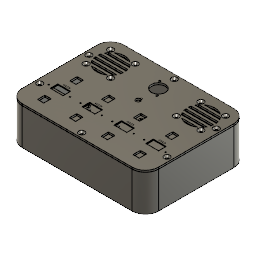
basestation_v3 (Autodesk Fusion 360 design; units mm, degrees)
Autodesk Fusion 360 part; units mm, degrees
note: some values were not read from the file. Chosen so that the rebuilt part matches the saved one: which face or edge a step refers to. Set by a fixed rule: which sketch regions a step uses.
(part 1 of 2)
sketch "Enclosure_main" plane through (0, 0, 0) normal (0, 1, 0) x (1, 0, 0)
  line L0 (0, 0) -> (230, 0)
  line L1 (230, 0) -> (230, -170)
  line L2 (230, -170) -> (0, -170)
  line L3 (0, -170) -> (0, 0)
  line L4 (0, -80) -> (10, -80)
  line L5 (10, -80) -> (10, -90)
  line L6 (10, -90) -> (0, -90)
  line L7 (0, -90) -> (0, -80)
  line L8 (0, -85) -> (230, -85) construction
  line L9 (115, 0) -> (115, -170) construction
  line L10 (5, -80) -> (5, -90) construction
  line L11 (0, -85) -> (10, -85) construction
  circle A0 centre (5, -85) radius 2.3
  line L12 (110, -10) -> (120, -10)
  line L13 (120, -10) -> (120, 0)
  line L14 (120, 0) -> (110, 0)
  line L15 (110, 0) -> (110, -10)
  line L16 (110, -5) -> (120, -5) construction
  line L17 (115, 0) -> (115, -10) construction
  circle A1 centre (115, -5) radius 2.3
  line L18 (220, -90) -> (230, -90)
  line L19 (230, -90) -> (230, -80)
  line L20 (230, -80) -> (220, -80)
  line L21 (220, -80) -> (220, -90)
  line L22 (225, -80) -> (225, -90) construction
  line L23 (220, -85) -> (230, -85) construction
  circle A2 centre (225, -85) radius 2.3
  line L24 (110, -170) -> (120, -170)
  line L25 (120, -170) -> (120, -160)
  line L26 (120, -160) -> (110, -160)
  line L27 (110, -160) -> (110, -170)
  line L28 (110, -165) -> (120, -165) construction
  line L29 (115, -170) -> (115, -160) construction
  circle A3 centre (115, -165) radius 2.3
  line L30 (20, -0.5) -> (76, -0.5) construction
  line L31 (76, -0.5) -> (76, -85.5) construction
  line L32 (76, -85.5) -> (20, -85.5) construction
  line L33 (20, -85.5) -> (20, -0.5) construction
  circle A4 centre (23.15, -3.65) radius 3
  circle A5 centre (23.15, -3.65) radius 1
  circle A6 centre (72.85, -3.65) radius 3
  circle A7 centre (72.85, -3.65) radius 1
  circle A8 centre (23.15, -61.65) radius 3
  circle A9 centre (72.85, -61.65) radius 3
  circle A10 centre (72.85, -61.65) radius 1
  circle A11 centre (23.15, -61.65) radius 1
  line L34 (181.9, -5) -> (181.9, -50) construction
  line L35 (181.9, -50) -> (151, -50) construction
  line L36 (151, -50) -> (151, -5) construction
  line L37 (151, -5) -> (181.9, -5) construction
  circle A12 centre (178.45, -46.55) radius 3
  circle A13 centre (154.45, -46.55) radius 3
  circle A14 centre (166.45, -10.3) radius 3
  circle A15 centre (166.45, -10.3) radius 1
  circle A16 centre (154.45, -46.55) radius 1
  circle A17 centre (178.45, -46.55) radius 1
  line L38 (79, -5) -> (99, -5) construction
  line L39 (99, -5) -> (99, -40) construction
  line L40 (99, -40) -> (79, -40) construction
  line L41 (79, -40) -> (79, -5) construction
  circle A18 centre (89, -8.9) radius 3
  circle A19 centre (89, -36.1) radius 3
  circle A20 centre (89, -36.1) radius 1
  circle A21 centre (89, -8.9) radius 1
  line L42 (78, -44.9949) -> (99.6, -45.0051) construction
  line L43 (99.6, -45.0051) -> (99.561, -75.7193) construction
  line L44 (99.561, -75.7193) -> (78, -76.2949) construction
  line L45 (78, -76.2949) -> (78, -44.9949) construction
  line L46 (88.8, -45) -> (88.7805, -76.0071) construction
  circle A22 centre (88.782, -73.6571) radius 3
  circle A23 centre (88.7985, -47.35) radius 3
  circle A24 centre (88.782, -73.6571) radius 1
  circle A25 centre (88.7985, -47.35) radius 1
  line L47 (166.45, -5) -> (166.45, -50) construction
  line L48 (0, -37.5) -> (10, -37.5)
  line L49 (10, -37.5) -> (10, -47.5)
  line L50 (10, -47.5) -> (0, -47.5)
  line L51 (0, -47.5) -> (0, -37.5)
  line L52 (0, -42.5) -> (10, -42.5) construction
  line L53 (5, -37.5) -> (5, -47.5) construction
  circle A26 centre (5, -42.5) radius 2.3
  line L54 (0, -122.5) -> (10, -122.5)
  line L55 (10, -122.5) -> (10, -132.5)
  line L56 (10, -132.5) -> (0, -132.5)
  line L57 (0, -132.5) -> (0, -122.5)
  line L58 (0, -127.5) -> (10, -127.5) construction
  line L59 (5, -122.5) -> (5, -132.5) construction
  circle A27 centre (5, -127.5) radius 2.3
  line L60 (220, -122.5) -> (230, -122.5)
  line L61 (230, -122.5) -> (230, -132.5)
  line L62 (230, -132.5) -> (220, -132.5)
  line L63 (220, -132.5) -> (220, -122.5)
  line L64 (220, -127.5) -> (230, -127.5) construction
  line L65 (225, -122.5) -> (225, -132.5) construction
  circle A28 centre (225, -127.5) radius 2.3
  line L66 (220, -37.5) -> (230, -37.5)
  line L67 (230, -37.5) -> (230, -47.5)
  line L68 (230, -47.5) -> (220, -47.5)
  line L69 (220, -47.5) -> (220, -37.5)
  line L70 (220, -42.5) -> (230, -42.5) construction
  line L71 (225, -37.5) -> (225, -47.5) construction
  circle A29 centre (225, -42.5) radius 2.3
  dimension "d1" = 170
  dimension "d2" = 230
  dimension "d282" = 10
  dimension "d283" = 10
  dimension "d284" = 4.6
  dimension "d307" = 10
  dimension "d308" = 10
  dimension "d309" = 4.6
  dimension "d310" = 10
  dimension "d311" = 10
  dimension "d312" = 4.6
  dimension "d313" = 10
  dimension "d314" = 10
  dimension "d315" = 4.6
  dimension "d349" = 56
  dimension "d350" = 85
  dimension "d351" = 20
  dimension "d352" = 0.5
  dimension "d353" = 6
  dimension "d354" = 2
  dimension "d355" = 3.15
  dimension "d356" = 3.15
  dimension "d357" = 6
  dimension "d358" = 3.15
  dimension "d359" = 3.15
  dimension "d360" = 2
  dimension "d361" = 6
  dimension "d362" = 3.15
  dimension "d363" = 58
  dimension "d364" = 6
  dimension "d365" = 3.15
  dimension "d366" = 58
  dimension "d367" = 2
  dimension "d368" = 2
  dimension "d369" = 45
  dimension "d370" = 30.9
  dimension "d371" = 6
  dimension "d372" = 6
  dimension "d373" = 6
  dimension "d375" = 3.45
  dimension "d376" = 3.45
  dimension "d377" = 3.45
  dimension "d378" = 3.45
  dimension "d379" = 2
  dimension "d380" = 2
  dimension "d381" = 2
  dimension "d384" = 20
  dimension "d385" = 35
  dimension "d386" = 6
  dimension "d387" = 10
  dimension "d388" = 3.9
  dimension "d389" = 6
  dimension "d390" = 10
  dimension "d391" = 3.9
  dimension "d392" = 2
  dimension "d393" = 2
  dimension "d394" = 5
  dimension "d395" = 3
  dimension "d396" = 21.6
  dimension "d397" = 31.3
  dimension "d398" = 6
  dimension "d399" = 6
  dimension "d402" = 2
  dimension "d403" = 2
  dimension "d469" = 5
  dimension "d470" = 75
  dimension "d471" = 5.3
  dimension "d484" = 10
  dimension "d485" = 10
  dimension "d486" = 4.6
  dimension "d487" = 42.5
  dimension "d488" = 10
  dimension "d489" = 10
  dimension "d490" = 4.6
  dimension "d491" = 42.5
  dimension "d492" = 10
  dimension "d493" = 10
  dimension "d494" = 4.6
  dimension "d495" = 42.5
  dimension "d496" = 10
  dimension "d497" = 10
  dimension "d498" = 42.5
  dimension "d499" = 4.6
  dimension "d517" = 2
  dimension "d518" = 2.35
  dimension "d519" = 2.35
  dimension "d520" = 5
  measures "d282" distance of L0.start
  measures "d284" diameter of A0
  measures "d308" distance of L0.start
  measures "d309" diameter of A1
  measures "d312" diameter of A2
  measures "d315" diameter of A3
  measures "d351" distance of L3 L33
  measures "d352" distance of L0 L30
  measures "d353" diameter of A4
  measures "d354" diameter of A5
  measures "d357" diameter of A6
  measures "d360" diameter of A7
  measures "d361" diameter of A8
  measures "d363" distance of L0.start
  measures "d364" diameter of A9
  measures "d366" distance of L0.start
  measures "d367" diameter of A10
  measures "d368" diameter of A11
  measures "d371" diameter of A12
  measures "d372" diameter of A13
  measures "d373" diameter of A14
  measures "d376" distance of L36 L0.start
  measures "d377" distance of L35 L3.end L0
  measures "d378" distance of L34 L3.end L0
  measures "d379" diameter of A15
  measures "d380" diameter of A16
  measures "d381" diameter of A17
  measures "d385" distance of L0.start
  measures "d386" diameter of A18
  measures "d387" distance of L41
  measures "d388" distance of L38
  measures "d389" diameter of A19
  measures "d390" distance of L41 L0.start
  measures "d392" diameter of A20
  measures "d393" diameter of A21
  measures "d394" distance of L0 L38
  measures "d395" distance of L31 L41
  measures "d398" diameter of A22
  measures "d399" diameter of A23
  measures "d402" diameter of A24 L1
  measures "d403" diameter of A25
  measures "d469" distance of L0 L37
  measures "d470" distance of L31 L36
  measures "d484" distance of L0.start
  measures "d486" diameter of A26
  measures "d488" distance of L0.start
  measures "d490" diameter of A27
  measures "d494" diameter of A28
  measures "d497" distance of L3.end origin L0
  measures "d499" diameter of A29
  measures "d517" distance of L31 L45
extrude "Extrude1" add sketch "Enclosure_main" along normal blind 60 contours L0 L1 L2 L3 L4 L5 L6 L12 L13 L15 L18 L20 L21 L25 L26 L27 L48 L49 L50 L54 L55 L56 L60 L62 L63 L66 L68 L69 | L0 L12 L13 L14 L15 | L3 L48 L49 L50 L51 | L3 L4 L5 L6 L7 | L1 L66 L67 L68 L69 | L3 L54 L55 L56 L57 | L1 L18 L19 L20 L21 | L1 L60 L61 L62 L63 | L2 L24 L25 L26 L27 | A0 | A1 | A2 | A3 | A4 | A5 | A6 | A7 | A8 | A9 | A10 | A11 | A12 | A13 | A14 | A15 | A16 | A17 | A18 | A19 | A20 | A21 | A22 | A23 | A24 | A25 | A26 | A27 | A28 | A29 makes body 1
fillet "Fillet1" radius 20 4 edges at (230, 30, 170) (0, 30, 170) (230, 30, 0) (0, 30, 0) on bodies 1
shell "Shell1" thickness 3 outward yes removed faces 0 bodies 1
ref_plane "WorkPlane1" through (115, 60, 85) normal (0, 1, 0) x (0, 0, 1)
split "Split1" by plane through (115, 60, 85) normal (0, 1, 0) bodies 1 makes body 2 at (83.3333, 63, 114.3333)
sketch "Enclosure_upper" plane through (0, 63, 0) normal (0, 1, 0) x (-1, 0, 0)
  arc A0 (-20, -3) -> (3, 20) centre (-20, 20) ccw
  line L0 (3, 20) -> (3, 150)
  arc A1 (3, 150) -> (-20, 173) centre (-20, 150) ccw
  line L1 (-20, 173) -> (-210, 173)
  arc A2 (-210, 173) -> (-233, 150) centre (-210, 150) ccw
  line L2 (-233, 150) -> (-233, 20)
  arc A3 (-233, 20) -> (-210, -3) centre (-210, 20) ccw
  line L3 (-210, -3) -> (-20, -3)
  line L4 (3, 85) -> (-233, 85) construction
  line L5 (-115, -3) -> (-115, 173) construction
  line L6 (-10.25, 10.25) -> (-63.75, 10.25) construction
  line L7 (-63.75, 10.25) -> (-63.75, 63.75) construction
  line L8 (-63.75, 63.75) -> (-10.25, 63.75) construction
  line L9 (-10.25, 63.75) -> (-10.25, 10.25) construction
  line L10 (-37, 10.25) -> (-37, 63.75) construction
  line L11 (-10.25, 37) -> (-63.75, 37) construction
  circle A4 centre (-37, 37) radius 24
  circle A5 centre (-15.75, 15.75) radius 2
  circle A6 centre (-58.25, 15.75) radius 2
  circle A7 centre (-58.25, 58.25) radius 2
  circle A8 centre (-15.75, 58.25) radius 2
  line L12 (-10.25, 13) -> (-63.75, 13)
  line L13 (-63.75, 13) -> (-63.75, 17.8)
  line L14 (-63.75, 17.8) -> (-10.25, 17.8)
  line L15 (-10.25, 17.8) -> (-10.25, 13)
  line L16 (-10.25, 17.8) -> (-63.75, 17.8)
  line L17 (-166.25, 13) -> (-219.75, 13)
  circle A9 centre (-171.75, 15.75) radius 2
  line L18 (-219.75, 17.8) -> (-166.25, 17.8)
  line L19 (-219.75, 13) -> (-219.75, 17.8)
  line L20 (-166.25, 17.8) -> (-219.75, 17.8)
  circle A10 centre (-214.25, 58.25) radius 2
  circle A11 centre (-171.75, 58.25) radius 2
  circle A12 centre (-214.25, 15.75) radius 2
  line L21 (-166.25, 17.8) -> (-166.25, 13)
  line L22 (-219.75, 10.25) -> (-219.75, 63.75) construction
  line L23 (-219.75, 63.75) -> (-166.25, 63.75) construction
  line L24 (-166.25, 10.25) -> (-219.75, 10.25) construction
  circle A13 centre (-193, 37) radius 24
  line L25 (-166.25, 63.75) -> (-166.25, 10.25) construction
  line L26 (-193, 10.25) -> (-193, 63.75) construction
  line L27 (-102, 17) -> (-128, 17) construction
  line L28 (-128, 17) -> (-128, 48) construction
  line L29 (-128, 48) -> (-102, 48) construction
  line L30 (-102, 48) -> (-102, 17) construction
  line L31 (-102, 32.5) -> (-128, 32.5) construction
  line L32 (-115, 17) -> (-115, 48) construction
  circle A14 centre (-115, 32.5) radius 12.15
  circle A15 centre (-105.2, 20.4) radius 1.6
  circle A16 centre (-124.8, 44.6) radius 1.6
  circle A17 centre (-115, 67.5) radius 5.75 construction
  circle A18 centre (-115, 67.5) radius 4
  line L33 (-113.5, 60.75) -> (-116.5, 60.75)
  line L34 (-116.5, 60.75) -> (-116.5, 62.75)
  line L35 (-116.5, 62.75) -> (-113.5, 62.75)
  line L36 (-113.5, 62.75) -> (-113.5, 60.75)
  line L37 (-113.5, 61.75) -> (-116.5, 61.75) construction
  line L38 (-115, 62.75) -> (-115, 60.75) construction
  line L39 (-10.25, 22.12) -> (-63.75, 22.12)
  line L40 (-10.25, 17.32) -> (-63.75, 17.32)
  line L41 (-10.25, 26.44) -> (-63.75, 26.44)
  line L42 (-10.25, 21.64) -> (-63.75, 21.64)
  line L43 (-10.25, 30.76) -> (-63.75, 30.76)
  line L44 (-10.25, 25.96) -> (-63.75, 25.96)
  line L45 (-10.25, 35.08) -> (-63.75, 35.08)
  line L46 (-10.25, 30.28) -> (-63.75, 30.28)
  line L47 (-10.25, 39.4) -> (-63.75, 39.4)
  line L48 (-10.25, 34.6) -> (-63.75, 34.6)
  line L49 (-10.25, 43.72) -> (-63.75, 43.72)
  line L50 (-10.25, 38.92) -> (-63.75, 38.92)
  line L51 (-10.25, 48.04) -> (-63.75, 48.04)
  line L52 (-10.25, 43.24) -> (-63.75, 43.24)
  line L53 (-10.25, 52.36) -> (-63.75, 52.36)
  line L54 (-10.25, 47.56) -> (-63.75, 47.56)
  line L55 (-10.25, 56.68) -> (-63.75, 56.68)
  line L56 (-10.25, 51.88) -> (-63.75, 51.88)
  line L57 (-10.25, 61) -> (-63.75, 61)
  line L58 (-10.25, 56.2) -> (-63.75, 56.2)
  line L59 (-166.25, 37) -> (-219.75, 37) construction
  line L60 (-166.25, 22.12) -> (-219.75, 22.12)
  line L61 (-166.25, 17.32) -> (-219.75, 17.32)
  line L62 (-166.25, 26.44) -> (-219.75, 26.44)
  line L63 (-166.25, 21.64) -> (-219.75, 21.64)
  line L64 (-166.25, 30.76) -> (-219.75, 30.76)
  line L65 (-166.25, 25.96) -> (-219.75, 25.96)
  line L66 (-166.25, 35.08) -> (-219.75, 35.08)
  line L67 (-166.25, 30.28) -> (-219.75, 30.28)
  line L68 (-166.25, 39.4) -> (-219.75, 39.4)
  line L69 (-166.25, 34.6) -> (-219.75, 34.6)
  line L70 (-166.25, 43.72) -> (-219.75, 43.72)
  line L71 (-166.25, 38.92) -> (-219.75, 38.92)
  line L72 (-166.25, 48.04) -> (-219.75, 48.04)
  line L73 (-166.25, 43.24) -> (-219.75, 43.24)
  line L74 (-166.25, 52.36) -> (-219.75, 52.36)
  line L75 (-166.25, 47.56) -> (-219.75, 47.56)
  line L76 (-166.25, 56.68) -> (-219.75, 56.68)
  line L77 (-166.25, 51.88) -> (-219.75, 51.88)
  line L78 (-166.25, 61) -> (-219.75, 61)
  line L79 (-166.25, 56.2) -> (-219.75, 56.2)
  line L80 (-27.15, 85) -> (-37.85, 85)
  line L81 (-37.85, 85) -> (-37.85, 97.7)
  line L82 (-37.85, 97.7) -> (-27.15, 97.7)
  line L83 (-27.15, 97.7) -> (-27.15, 85)
  line L84 (-27.15, 91.35) -> (-37.85, 91.35) construction
  line L85 (-32.5, 85) -> (-32.5, 97.7) construction
  line L86 (-18.5, 106.9) -> (-46.5, 106.9)
  line L87 (-46.5, 106.9) -> (-46.5, 135.4)
  line L88 (-46.5, 135.4) -> (-18.5, 135.4)
  line L89 (-18.5, 135.4) -> (-18.5, 106.9)
  line L90 (-18.5, 121.15) -> (-46.5, 121.15) construction
  line L91 (-32.5, 106.9) -> (-32.5, 135.4) construction
  line L92 (-21.5, 112.7) -> (-43.5, 112.7)
  line L93 (-43.5, 112.7) -> (-43.5, 125.7)
  line L94 (-43.5, 125.7) -> (-21.5, 125.7)
  line L95 (-21.5, 125.7) -> (-21.5, 112.7)
  line L96 (-27.15, 140.7) -> (-37.85, 140.7)
  line L97 (-37.85, 140.7) -> (-37.85, 153.4)
  line L98 (-37.85, 153.4) -> (-27.15, 153.4)
  line L99 (-27.15, 153.4) -> (-27.15, 140.7)
  line L100 (-32.5, 140.7) -> (-32.5, 153.4) construction
  line L101 (-27.15, 147.05) -> (-37.7784, 147.05) construction
  line L102 (-47, 117.25) -> (-54.8, 117.25)
  line L103 (-54.8, 117.25) -> (-54.8, 125.05)
  line L104 (-54.8, 125.05) -> (-47, 125.05)
  line L105 (-47, 125.05) -> (-47, 117.25)
  line L106 (-50.9, 117.25) -> (-50.9, 125.05) construction
  line L107 (-54.8, 121.15) -> (-47, 121.15) construction
  circle A19 centre (-50.9, 121.15) radius 1.6
  circle A20 centre (-50.9, 121.15) radius 1
  line L108 (-18, 117.25) -> (-10.2, 117.25)
  line L109 (-10.2, 117.25) -> (-10.2, 125.05)
  line L110 (-10.2, 125.05) -> (-18, 125.05)
  line L111 (-18, 125.05) -> (-18, 117.25)
  line L112 (-14.1, 117.25) -> (-14.1, 125.05) construction
  line L113 (-10.2, 121.15) -> (-18, 121.15) construction
  circle A21 centre (-14.1, 121.15) radius 1.6
  circle A22 centre (-14.1, 121.15) radius 1
  line L114 (-19, 107.4) -> (-24.5, 107.4)
  line L115 (-24.5, 107.4) -> (-24.5, 110.15)
  line L116 (-24.5, 110.15) -> (-19, 110.15)
  line L117 (-19, 110.15) -> (-19, 107.4)
  line L118 (-40.5, 107.4) -> (-46, 107.4)
  line L119 (-46, 107.4) -> (-46, 110.15)
  line L120 (-46, 110.15) -> (-40.5, 110.15)
  line L121 (-40.5, 110.15) -> (-40.5, 107.4)
  line L122 (-27.15, 107.4) -> (-37.85, 107.4)
  line L123 (-37.85, 107.4) -> (-37.85, 109.4)
  line L124 (-37.85, 109.4) -> (-27.15, 109.4)
  line L125 (-27.15, 109.4) -> (-27.15, 107.4)
  line L126 (-40.5, 132.15) -> (-46, 132.15)
  line L127 (-46, 132.15) -> (-46, 134.9)
  line L128 (-46, 134.9) -> (-40.5, 134.9)
  line L129 (-40.5, 134.9) -> (-40.5, 132.15)
  line L130 (-19, 132.15) -> (-24.5, 132.15)
  line L131 (-24.5, 132.15) -> (-24.5, 134.9)
  line L132 (-24.5, 134.9) -> (-19, 134.9)
  line L133 (-19, 134.9) -> (-19, 132.15)
  line L134 (-10.2, 117.25) -> (-54.8, 117.25)
  line L135 (-54.8, 117.25) -> (-54.8, 125.05)
  line L136 (-54.8, 125.05) -> (-10.2, 125.05)
  line L137 (-10.2, 125.05) -> (-10.2, 117.25)
  line L138 (-65.2, 125.05) -> (-73, 125.05)
  line L139 (-82.15, 91.35) -> (-92.85, 91.35) construction
  line L140 (-82.15, 107.4) -> (-92.85, 107.4)
  line L141 (-98.5, 125.7) -> (-76.5, 125.7)
  line L142 (-92.85, 85) -> (-92.85, 97.7)
  line L143 (-92.85, 107.4) -> (-92.85, 109.4)
  line L144 (-82.15, 109.4) -> (-82.15, 107.4)
  line L145 (-105.9, 117.25) -> (-105.9, 125.05) construction
  line L146 (-76.5, 125.7) -> (-76.5, 112.7)
  circle A23 centre (-105.9, 121.15) radius 1
  line L147 (-79.5, 134.9) -> (-74, 134.9)
  line L148 (-73, 117.25) -> (-65.2, 117.25)
  line L149 (-65.2, 117.25) -> (-65.2, 125.05)
  line L150 (-69.1, 117.25) -> (-69.1, 125.05) construction
  line L151 (-102, 117.25) -> (-109.8, 117.25)
  line L152 (-102, 125.05) -> (-102, 117.25)
  circle A24 centre (-105.9, 121.15) radius 1.6
  line L153 (-74, 132.15) -> (-79.5, 132.15)
  circle A25 centre (-69.1, 121.15) radius 1
  line L154 (-65.2, 125.05) -> (-65.2, 117.25)
  line L155 (-73, 125.05) -> (-73, 117.25)
  line L156 (-74, 134.9) -> (-74, 132.15)
  line L157 (-87.5, 85) -> (-87.5, 97.7) construction
  line L158 (-79.5, 110.15) -> (-74, 110.15)
  line L159 (-92.85, 109.4) -> (-82.15, 109.4)
  line L160 (-79.5, 132.15) -> (-79.5, 134.9)
  line L161 (-65.2, 121.15) -> (-73, 121.15) construction
  circle A26 centre (-69.1, 121.15) radius 1.6
  line L162 (-95.5, 132.15) -> (-101, 132.15)
  line L163 (-95.5, 134.9) -> (-95.5, 132.15)
  line L164 (-109.8, 121.15) -> (-102, 121.15) construction
  line L165 (-109.8, 125.05) -> (-102, 125.05)
  line L166 (-65.2, 117.25) -> (-109.8, 117.25)
  line L167 (-87.5, 106.9) -> (-87.5, 135.4) construction
  line L168 (-95.5, 107.4) -> (-101, 107.4)
  line L169 (-82.15, 140.7) -> (-92.85, 140.7)
  line L170 (-101, 107.4) -> (-101, 110.15)
  line L171 (-101, 110.15) -> (-95.5, 110.15)
  line L172 (-73, 106.4) -> (-102, 106.4)
  line L173 (-76.5, 112.7) -> (-98.5, 112.7)
  line L174 (-74, 107.4) -> (-79.5, 107.4)
  line L175 (-98.5, 112.7) -> (-98.5, 125.7)
  line L176 (-95.5, 110.15) -> (-95.5, 107.4)
  line L177 (-79.5, 107.4) -> (-79.5, 110.15)
  line L178 (-73, 135.9) -> (-73, 106.4)
  line L179 (-102, 135.9) -> (-73, 135.9)
  line L180 (-82.15, 153.4) -> (-82.15, 140.7)
  line L181 (-82.15, 147.05) -> (-92.7784, 147.05) construction
  line L182 (-73.5, 121.15) -> (-101.5, 121.15) construction
  line L183 (-92.85, 153.4) -> (-82.15, 153.4)
  line L184 (-101.5, 135.4) -> (-73.5, 135.4)
  line L185 (-73.5, 106.9) -> (-101.5, 106.9)
  line L186 (-92.85, 140.7) -> (-92.85, 153.4)
  line L187 (-87.5, 140.7) -> (-87.5, 153.4) construction
  line L188 (-109.8, 125.05) -> (-65.2, 125.05)
  line L189 (-73.5, 135.4) -> (-73.5, 106.9)
  line L190 (-102, 106.4) -> (-102, 135.9)
  line L191 (-101.5, 106.9) -> (-101.5, 135.4)
  line L192 (-109.8, 117.25) -> (-109.8, 125.05)
  line L193 (-109.8, 117.25) -> (-109.8, 125.05)
  line L194 (-74, 110.15) -> (-74, 107.4)
  line L195 (-82.15, 85) -> (-92.85, 85)
  line L196 (-101, 134.9) -> (-95.5, 134.9)
  line L197 (-82.15, 97.7) -> (-82.15, 85)
  line L198 (-92.85, 97.7) -> (-82.15, 97.7)
  line L199 (-101, 132.15) -> (-101, 134.9)
  line L200 (-137.15, 91.35) -> (-147.85, 91.35) construction
  line L201 (-156, 110.15) -> (-150.5, 110.15)
  line L202 (-131.5, 125.7) -> (-131.5, 112.7)
  line L203 (-147.85, 97.7) -> (-137.15, 97.7)
  line L204 (-128, 117.25) -> (-120.2, 117.25)
  line L205 (-137.15, 97.7) -> (-137.15, 85)
  line L206 (-137.15, 107.4) -> (-147.85, 107.4)
  line L207 (-147.85, 107.4) -> (-147.85, 109.4)
  line L208 (-147.85, 109.4) -> (-137.15, 109.4)
  line L209 (-147.85, 153.4) -> (-137.15, 153.4)
  line L210 (-142.5, 140.7) -> (-142.5, 153.4) construction
  line L211 (-150.5, 134.9) -> (-150.5, 132.15)
  line L212 (-150.5, 132.15) -> (-156, 132.15)
  line L213 (-147.85, 85) -> (-147.85, 97.7)
  line L214 (-142.5, 106.9) -> (-142.5, 135.4) construction
  line L215 (-120.2, 117.25) -> (-120.2, 125.05)
  line L216 (-128, 135.9) -> (-128, 106.4)
  line L217 (-150.5, 107.4) -> (-156, 107.4)
  line L218 (-137.15, 85) -> (-147.85, 85)
  line L219 (-150.5, 110.15) -> (-150.5, 107.4)
  line L220 (-128.5, 121.15) -> (-156.5, 121.15) construction
  line L221 (-156.5, 135.4) -> (-128.5, 135.4)
  line L222 (-147.85, 140.7) -> (-147.85, 153.4)
  line L223 (-153.5, 112.7) -> (-153.5, 125.7)
  line L224 (-128.5, 135.4) -> (-128.5, 106.9)
  line L225 (-156, 134.9) -> (-150.5, 134.9)
  line L226 (-142.5, 85) -> (-142.5, 97.7) construction
  line L227 (-124.1, 117.25) -> (-124.1, 125.05) construction
  line L228 (-134.5, 134.9) -> (-129, 134.9)
  line L229 (-164.8, 125.05) -> (-120.2, 125.05)
  line L230 (-128.5, 106.9) -> (-156.5, 106.9)
  line L231 (-120.2, 125.05) -> (-128, 125.05)
  line L232 (-157, 106.4) -> (-157, 135.9)
  line L233 (-156, 132.15) -> (-156, 134.9)
  line L234 (-164.8, 117.25) -> (-164.8, 125.05)
  line L235 (-164.8, 125.05) -> (-157, 125.05)
  line L236 (-164.8, 121.15) -> (-157, 121.15) construction
  line L237 (-120.2, 117.25) -> (-164.8, 117.25)
  line L238 (-153.5, 125.7) -> (-131.5, 125.7)
  line L239 (-160.9, 117.25) -> (-160.9, 125.05) construction
  line L240 (-137.15, 153.4) -> (-137.15, 140.7)
  line L241 (-128, 106.4) -> (-157, 106.4)
  line L242 (-137.15, 147.05) -> (-147.7784, 147.05) construction
  line L243 (-157, 135.9) -> (-128, 135.9)
  circle A27 centre (-160.9, 121.15) radius 1
  line L244 (-156, 107.4) -> (-156, 110.15)
  line L245 (-164.8, 117.25) -> (-164.8, 125.05)
  line L246 (-156.5, 106.9) -> (-156.5, 135.4)
  circle A28 centre (-160.9, 121.15) radius 1.6
  line L247 (-137.15, 140.7) -> (-147.85, 140.7)
  line L248 (-157, 117.25) -> (-164.8, 117.25)
  line L249 (-157, 125.05) -> (-157, 117.25)
  line L250 (-131.5, 112.7) -> (-153.5, 112.7)
  line L251 (-129, 134.9) -> (-129, 132.15)
  circle A29 centre (-124.1, 121.15) radius 1
  circle A30 centre (-124.1, 121.15) radius 1.6
  line L252 (-134.5, 110.15) -> (-129, 110.15)
  line L253 (-134.5, 107.4) -> (-134.5, 110.15)
  line L254 (-129, 107.4) -> (-134.5, 107.4)
  line L255 (-128, 125.05) -> (-128, 117.25)
  line L256 (-129, 110.15) -> (-129, 107.4)
  line L257 (-137.15, 109.4) -> (-137.15, 107.4)
  line L258 (-129, 132.15) -> (-134.5, 132.15)
  line L259 (-120.2, 125.05) -> (-120.2, 117.25)
  line L260 (-120.2, 121.15) -> (-128, 121.15) construction
  line L261 (-134.5, 132.15) -> (-134.5, 134.9)
  line L262 (-192.15, 91.35) -> (-202.85, 91.35) construction
  line L263 (-211, 110.15) -> (-205.5, 110.15)
  line L264 (-186.5, 125.7) -> (-186.5, 112.7)
  line L265 (-202.85, 97.7) -> (-192.15, 97.7)
  line L266 (-183, 117.25) -> (-175.2, 117.25)
  line L267 (-192.15, 97.7) -> (-192.15, 85)
  line L268 (-192.15, 107.4) -> (-202.85, 107.4)
  line L269 (-202.85, 107.4) -> (-202.85, 109.4)
  line L270 (-202.85, 109.4) -> (-192.15, 109.4)
  line L271 (-202.85, 153.4) -> (-192.15, 153.4)
  line L272 (-197.5, 140.7) -> (-197.5, 153.4) construction
  line L273 (-205.5, 134.9) -> (-205.5, 132.15)
  line L274 (-205.5, 132.15) -> (-211, 132.15)
  line L275 (-202.85, 85) -> (-202.85, 97.7)
  line L276 (-197.5, 106.9) -> (-197.5, 135.4) construction
  line L277 (-175.2, 117.25) -> (-175.2, 125.05)
  line L278 (-183, 135.9) -> (-183, 106.4)
  line L279 (-205.5, 107.4) -> (-211, 107.4)
  line L280 (-192.15, 85) -> (-202.85, 85)
  line L281 (-205.5, 110.15) -> (-205.5, 107.4)
  line L282 (-183.5, 121.15) -> (-211.5, 121.15) construction
  line L283 (-211.5, 135.4) -> (-183.5, 135.4)
  line L284 (-202.85, 140.7) -> (-202.85, 153.4)
  line L285 (-208.5, 112.7) -> (-208.5, 125.7)
  line L286 (-183.5, 135.4) -> (-183.5, 106.9)
  line L287 (-211, 134.9) -> (-205.5, 134.9)
  line L288 (-197.5, 85) -> (-197.5, 97.7) construction
  line L289 (-179.1, 117.25) -> (-179.1, 125.05) construction
  line L290 (-189.5, 134.9) -> (-184, 134.9)
  line L291 (-219.8, 125.05) -> (-175.2, 125.05)
  line L292 (-183.5, 106.9) -> (-211.5, 106.9)
  line L293 (-175.2, 125.05) -> (-183, 125.05)
  line L294 (-212, 106.4) -> (-212, 135.9)
  line L295 (-211, 132.15) -> (-211, 134.9)
  line L296 (-219.8, 117.25) -> (-219.8, 125.05)
  line L297 (-219.8, 125.05) -> (-212, 125.05)
  line L298 (-219.8, 121.15) -> (-212, 121.15) construction
  line L299 (-175.2, 117.25) -> (-219.8, 117.25)
  line L300 (-208.5, 125.7) -> (-186.5, 125.7)
  line L301 (-215.9, 117.25) -> (-215.9, 125.05) construction
  line L302 (-192.15, 153.4) -> (-192.15, 140.7)
  line L303 (-183, 106.4) -> (-212, 106.4)
  line L304 (-192.15, 147.05) -> (-202.7784, 147.05) construction
  line L305 (-212, 135.9) -> (-183, 135.9)
  circle A31 centre (-215.9, 121.15) radius 1
  line L306 (-211, 107.4) -> (-211, 110.15)
  line L307 (-219.8, 117.25) -> (-219.8, 125.05)
  line L308 (-211.5, 106.9) -> (-211.5, 135.4)
  circle A32 centre (-215.9, 121.15) radius 1.6
  line L309 (-192.15, 140.7) -> (-202.85, 140.7)
  line L310 (-212, 117.25) -> (-219.8, 117.25)
  line L311 (-212, 125.05) -> (-212, 117.25)
  line L312 (-186.5, 112.7) -> (-208.5, 112.7)
  line L313 (-184, 134.9) -> (-184, 132.15)
  circle A33 centre (-179.1, 121.15) radius 1
  circle A34 centre (-179.1, 121.15) radius 1.6
  line L314 (-189.5, 110.15) -> (-184, 110.15)
  line L315 (-189.5, 107.4) -> (-189.5, 110.15)
  line L316 (-184, 107.4) -> (-189.5, 107.4)
  line L317 (-183, 125.05) -> (-183, 117.25)
  line L318 (-184, 110.15) -> (-184, 107.4)
  line L319 (-192.15, 109.4) -> (-192.15, 107.4)
  line L320 (-184, 132.15) -> (-189.5, 132.15)
  line L321 (-175.2, 125.05) -> (-175.2, 117.25)
  line L322 (-175.2, 121.15) -> (-183, 121.15) construction
  line L323 (-189.5, 132.15) -> (-189.5, 134.9)
  line L324 (-7, 70.75) -> (-19, 70.75)
  line L325 (-19, 70.75) -> (-19, 75.75)
  line L326 (-19, 75.75) -> (-7, 75.75)
  line L327 (-7, 75.75) -> (-7, 70.75)
  line L328 (0, 92.5) -> (-2.5, 92.5)
  line L329 (-2.5, 92.5) -> (-2.5, 77.5)
  line L330 (-2.5, 77.5) -> (0, 77.5)
  line L331 (0, 77.5) -> (0, 92.5)
  circle A35 centre (-115, 5) radius 2
  circle A36 centre (-115, 165) radius 2
  line L332 (-107.5, 2.5) -> (-122.5, 2.5)
  line L333 (-122.5, 2.5) -> (-122.5, 0)
  line L334 (-122.5, 0) -> (-107.5, 0)
  line L335 (-107.5, 0) -> (-107.5, 2.5)
  line L336 (-227.5, 92.5) -> (-230, 92.5)
  line L337 (-230, 92.5) -> (-230, 77.5)
  line L338 (-230, 77.5) -> (-227.5, 77.5)
  line L339 (-227.5, 77.5) -> (-227.5, 92.5)
  line L340 (-107.5, 170) -> (-122.5, 170)
  line L341 (-122.5, 170) -> (-122.5, 167.5)
  line L342 (-122.5, 167.5) -> (-107.5, 167.5)
  line L343 (-107.5, 167.5) -> (-107.5, 170)
  line L344 (-20, 169.5) -> (-210, 169.5)
  arc A37 (-210, 169.5) -> (-229.5, 150) centre (-210, 150) ccw
  line L345 (-229.5, 150) -> (-229.5, 20)
  arc A38 (-229.5, 20) -> (-210, 0.5) centre (-210, 20) ccw
  line L346 (-210, 0.5) -> (-20, 0.5)
  arc A39 (-20, 0.5) -> (-0.5, 20) centre (-20, 20) ccw
  line L347 (-0.5, 20) -> (-0.5, 150)
  arc A40 (-0.5, 150) -> (-20, 169.5) centre (-20, 150) ccw
  line L348 (-20, 168) -> (-210, 168)
  arc A41 (-210, 168) -> (-228, 150) centre (-210, 150) ccw
  line L349 (-228, 150) -> (-228, 20)
  arc A42 (-228, 20) -> (-210, 2) centre (-210, 20) ccw
  line L350 (-210, 2) -> (-20, 2)
  arc A43 (-20, 2) -> (-2, 20) centre (-20, 20) ccw
  line L351 (-2, 20) -> (-2, 150)
  arc A44 (-2, 150) -> (-20, 168) centre (-20, 150) ccw
  line L352 (-47, 106.4) -> (-47, 135.9)
  line L353 (-47, 135.9) -> (-18, 135.9)
  line L354 (-18, 135.9) -> (-18, 106.4)
  line L355 (-18, 106.4) -> (-47, 106.4)
  circle A45 centre (-5, 42.5) radius 2
  circle A46 centre (-5, 127.5) radius 2
  circle A47 centre (-225, 127.5) radius 2
  circle A48 centre (-225, 42.5) radius 2
  line L356 (0, 135) -> (-2.5, 135)
  line L357 (-2.5, 135) -> (-2.5, 120)
  line L358 (-2.5, 120) -> (0, 120)
  line L359 (0, 120) -> (0, 135)
  line L360 (0, 50) -> (-2.5, 50)
  line L361 (-2.5, 50) -> (-2.5, 35)
  line L362 (-2.5, 35) -> (0, 35)
  line L363 (0, 35) -> (0, 50)
  line L364 (-227.5, 50) -> (-230, 50)
  line L365 (-230, 50) -> (-230, 35)
  line L366 (-230, 35) -> (-227.5, 35)
  line L367 (-227.5, 35) -> (-227.5, 50)
  line L368 (-227.5, 135) -> (-230, 135)
  line L369 (-230, 135) -> (-230, 120)
  line L370 (-230, 120) -> (-227.5, 120)
  line L371 (-227.5, 120) -> (-227.5, 135)
  point P0 (0, -20)
  dimension "d8" = 3.5
  dimension "d9" = 5
  dimension "d16" = 53.5
  dimension "d17" = 53.5
  dimension "d18" = 48
  dimension "d19" = 4
  dimension "d20" = 5.5
  dimension "d21" = 5.5
  dimension "d22" = 40
  dimension "d23" = 40
  dimension "d24" = 4
  dimension "d25" = 5.5
  dimension "d26" = 5.5
  dimension "d27" = 4
  dimension "d28" = 5.5
  dimension "d29" = 5.5
  dimension "d30" = 4
  dimension "d31" = 5.5
  dimension "d32" = 5.5
  dimension "d33" = 4.8
  dimension "d34" = 2.75
  dimension "d39" = 53.5
  dimension "d40" = 53.5
  dimension "d41" = 48
  dimension "d42" = 4
  dimension "d43" = 5.5
  dimension "d44" = 5.5
  dimension "d45" = 4
  dimension "d46" = 5.5
  dimension "d47" = 5.5
  dimension "d48" = 4
  dimension "d49" = 5.5
  dimension "d50" = 5.5
  dimension "d51" = 4
  dimension "d52" = 5.5
  dimension "d53" = 5.5
  dimension "d54" = 4.8
  dimension "d55" = 2.75
  dimension "d56" = 40
  dimension "d57" = 40
  dimension "d58" = 26
  dimension "d59" = 31
  dimension "d60" = 24.3
  dimension "d61" = 3.2
  dimension "d62" = 3.2
  dimension "d63" = 3.4
  dimension "d64" = 3.2
  dimension "d65" = 3.4
  dimension "d66" = 3.2
  dimension "d67" = 20
  dimension "d68" = 11.5
  dimension "d69" = 35
  dimension "d70" = 8
  dimension "d71" = 3
  dimension "d72" = 2
  dimension "d77" = 0
  dimension "d78" = 43.2
  dimension "d81" = 0
  dimension "d82" = 43.2
  dimension "d86" = 35.5
  dimension "d87" = 55
  dimension "d88" = 55
  dimension "d89" = 55
  dimension "d90" = 10.7
  dimension "d91" = 12.7
  dimension "d92" = 28
  dimension "d93" = 28.5
  dimension "d94" = 22
  dimension "d95" = 13
  dimension "d96" = 5.8
  dimension "d97" = 0.5
  dimension "d98" = 15
  dimension "d99" = 10.7
  dimension "d100" = 12.7
  dimension "d101" = 15
  dimension "d102" = 7.8
  dimension "d103" = 7.8
  dimension "d104" = 3.2
  dimension "d105" = 2
  dimension "d106" = 7.8
  dimension "d107" = 7.8
  dimension "d108" = 3.2
  dimension "d109" = 2
  dimension "d110" = 5.5
  dimension "d111" = 2.75
  dimension "d112" = 0.5
  dimension "d113" = 0.5
  dimension "d114" = 5.5
  dimension "d115" = 2.75
  dimension "d116" = 0.5
  dimension "d117" = 0.5
  dimension "d118" = 10.7
  dimension "d119" = 2
  dimension "d120" = 0.5
  dimension "d121" = 5.5
  dimension "d122" = 2.75
  dimension "d123" = 0.5
  dimension "d124" = 0.5
  dimension "d125" = 5.5
  dimension "d126" = 2.75
  dimension "d127" = 0.5
  dimension "d128" = 0.5
  dimension "d129" = 10.7
  dimension "d130" = 12.7
  dimension "d131" = 28
  dimension "d132" = 28.5
  dimension "d133" = 22
  dimension "d134" = 13
  dimension "d135" = 5.8
  dimension "d136" = 0.5
  dimension "d137" = 15
  dimension "d138" = 10.7
  dimension "d139" = 12.7
  dimension "d140" = 15
  dimension "d141" = 7.8
  dimension "d142" = 7.8
  dimension "d143" = 3.2
  dimension "d144" = 2
  dimension "d145" = 7.8
  dimension "d146" = 7.8
  dimension "d147" = 3.2
  dimension "d148" = 2
  dimension "d149" = 5.5
  dimension "d150" = 2.75
  dimension "d151" = 0.5
  dimension "d152" = 0.5
  dimension "d153" = 5.5
  dimension "d154" = 2.75
  dimension "d155" = 0.5
  dimension "d156" = 0.5
  dimension "d157" = 10.7
  dimension "d158" = 2
  dimension "d159" = 0.5
  dimension "d160" = 5.5
  dimension "d161" = 2.75
  dimension "d162" = 0.5
  dimension "d163" = 0.5
  dimension "d164" = 5.5
  dimension "d165" = 2.75
  dimension "d166" = 0.5
  dimension "d167" = 0.5
  dimension "d168" = 10.7
  dimension "d169" = 12.7
  dimension "d170" = 28
  dimension "d171" = 28.5
  dimension "d172" = 22
  dimension "d173" = 13
  dimension "d174" = 5.8
  dimension "d175" = 0.5
  dimension "d176" = 15
  dimension "d177" = 10.7
  dimension "d178" = 12.7
  dimension "d179" = 15
  dimension "d180" = 7.8
  dimension "d181" = 7.8
  dimension "d182" = 3.2
  dimension "d183" = 2
  dimension "d184" = 7.8
  dimension "d185" = 7.8
  dimension "d186" = 3.2
  dimension "d187" = 2
  dimension "d188" = 5.5
  dimension "d189" = 2.75
  dimension "d190" = 0.5
  dimension "d191" = 0.5
  dimension "d192" = 5.5
  dimension "d193" = 2.75
  dimension "d194" = 0.5
  dimension "d195" = 0.5
  dimension "d196" = 10.7
  dimension "d197" = 2
  dimension "d198" = 0.5
  dimension "d199" = 5.5
  dimension "d200" = 2.75
  dimension "d201" = 0.5
  dimension "d202" = 0.5
  dimension "d203" = 5.5
  dimension "d204" = 2.75
  dimension "d205" = 0.5
  dimension "d206" = 0.5
  dimension "d207" = 10.7
  dimension "d208" = 12.7
  dimension "d209" = 28
  dimension "d210" = 28.5
  dimension "d211" = 22
  dimension "d212" = 13
  dimension "d213" = 5.8
  dimension "d214" = 0.5
  dimension "d215" = 15
  dimension "d216" = 10.7
  dimension "d217" = 12.7
  dimension "d218" = 15
  dimension "d219" = 7.8
  dimension "d220" = 7.8
  dimension "d221" = 3.2
  dimension "d222" = 2
  dimension "d223" = 7.8
  dimension "d224" = 7.8
  dimension "d225" = 3.2
  dimension "d226" = 2
  dimension "d227" = 5.5
  dimension "d228" = 2.75
  dimension "d229" = 0.5
  dimension "d230" = 0.5
  dimension "d231" = 5.5
  dimension "d232" = 2.75
  dimension "d233" = 0.5
  dimension "d234" = 0.5
  dimension "d235" = 10.7
  dimension "d236" = 2
  dimension "d237" = 0.5
  dimension "d238" = 5.5
  dimension "d239" = 2.75
  dimension "d240" = 0.5
  dimension "d241" = 0.5
  dimension "d242" = 5.5
  dimension "d243" = 2.75
  dimension "d244" = 0.5
  dimension "d245" = 0.5
  dimension "d270" = 12
  dimension "d271" = 5
  dimension "d296" = 2.5
  dimension "d297" = 15
  dimension "d336" = 4
  dimension "d338" = 4
  dimension "d339" = 15
  dimension "d340" = 2.5
  dimension "d341" = 2.5
  dimension "d342" = 15
  dimension "d343" = 15
  dimension "d344" = 2.5
  dimension "d444" = 10
  dimension "d445" = 7
  dimension "d504" = 4
  dimension "d505" = 4
  dimension "d506" = 4
  dimension "d507" = 4
  dimension "d508" = 2.5
  dimension "d509" = 15
  dimension "d510" = 2.5
  dimension "d511" = 15
  dimension "d512" = 2.5
  dimension "d513" = 15
  dimension "d514" = 2.5
  dimension "d515" = 15
  measures "d18" diameter of A4
  measures "d19" diameter of A5
  measures "d20" distance of L6
  measures "d21" distance of L9
  measures "d22" distance of L3 origin
  measures "d23" distance of L0 origin
  measures "d24" diameter of A6
  measures "d25" distance of L6
  measures "d26" distance of L7
  measures "d27" diameter of A7
  measures "d28" distance of L8 origin
  measures "d29" distance of L7 origin
  measures "d30" diameter of A8
  measures "d31" distance of L9
  measures "d32" distance of L8
  measures "d34" distance of L6 L12
  measures "d40" distance of origin
  measures "d41" diameter of A13
  measures "d42" diameter of A9
  measures "d43" distance of L24
  measures "d44" distance of L25
  measures "d45" diameter of A12
  measures "d46" distance of L24
  measures "d47" distance of L22
  measures "d48" diameter of A10
  measures "d50" distance of origin L22
  measures "d51" diameter of A11
  measures "d52" distance of origin L25
  measures "d55" distance of L17 L24
  measures "d56" distance of L3 origin
  measures "d59" distance of origin
  measures "d60" diameter of A14
  measures "d61" diameter of A15
  measures "d62" distance of L30 origin
  measures "d63" distance of L27 origin
  measures "d64" diameter of A16
  measures "d66" distance of L28 origin
  measures "d68" diameter of A17
  measures "d70" diameter of A18
  measures "d86" distance of origin
  measures "d92" distance of origin
  measures "d96" distance of L86 L92
  measures "d104" diameter of A19
  measures "d105" diameter of A20
  measures "d108" diameter of A21
  measures "d109" diameter of A22
  measures "d110" distance of origin
  measures "d112" distance of L86 L114
  measures "d113" distance of L89 L117
  measures "d116" distance of L87 L119
  measures "d117" distance of L86 L118
  measures "d120" distance of L86 L122
  measures "d123" distance of L88 L128
  measures "d124" distance of L87 L127
  measures "d125" distance of origin
  measures "d127" distance of L88 L132
  measures "d128" distance of L89 L133
  measures "d135" distance of L173 L185
  measures "d143" diameter of A24
  measures "d144" diameter of A23
  measures "d147" diameter of A26
  measures "d148" diameter of A25
  measures "d151" distance of L174 L185
  measures "d152" distance of L189 L194
  measures "d155" distance of L170 L191
  measures "d156" distance of L168 L185
  measures "d159" distance of L140 L185
  measures "d162" distance of L184 L196
  measures "d163" distance of L191 L199
  measures "d166" distance of L147 L184
  measures "d167" distance of L156 L189
  measures "d174" distance of L230 L250
  measures "d182" diameter of A28
  measures "d183" diameter of A27
  measures "d186" diameter of A30
  measures "d187" diameter of A29
  measures "d190" distance of L230 L254
  measures "d191" distance of L224 L256
  measures "d194" distance of L244 L246
  measures "d195" distance of L217 L230
  measures "d198" distance of L206 L230
  measures "d201" distance of L221 L225
  measures "d202" distance of L233 L246
  measures "d205" distance of L221 L228
  measures "d206" distance of L224 L251
  measures "d213" distance of L292 L312
  measures "d221" diameter of A32
  measures "d222" diameter of A31
  measures "d225" diameter of A34
  measures "d226" diameter of A33
  measures "d229" distance of L292 L316
  measures "d230" distance of L286 L318
  measures "d233" distance of L306 L308
  measures "d234" distance of L279 L292
  measures "d237" distance of L268 L292
  measures "d240" distance of L283 L287
  measures "d241" distance of L295 L308
  measures "d244" distance of L283 L290
  measures "d245" distance of L286 L313
  measures "d296" distance of origin
  measures "d336" diameter of A35
  measures "d338" diameter of A36
  measures "d340" distance of origin
  measures "d444" distance of L0 L327
  measures "d445" distance of L8 L324
  measures "d504" diameter of A45
  measures "d505" diameter of A46
  measures "d506" diameter of A47
  measures "d507" diameter of A48
  measures "d508" distance of origin
  measures "d510" distance of origin
extrude "Extrude15" add sketch "Enclosure_main" against normal blind 18 from surface at 60 contours L0 L12 L13 L14 L15 | L3 L48 L49 L50 L51 | L1 L66 L67 L68 L69 | L3 L54 L55 L56 L57 | L1 L60 L61 L62 L63 | L2 L24 L25 L26 L27 | A1 | A3 | A26 | A27 | A28 | A29 bodies 1
extrude "Extrude16" cut sketch "Enclosure_main" against normal blind 18 from surface at 60 contours A1 | A3 | A26 | A27 | A28 | A29 bodies 1
chamfer "Chamfer4" distance 10 angle 45 6 edges at (10, 42, 42.5) (10, 42, 127.5) (115, 42, 10) (220, 42, 42.5) (220, 42, 127.5) (115, 42, 160) on bodies 1
fillet "Fillet7" radius 2 24 edges at (120, 51, 0) (120, 56, 10) (110, 56, 10) (110, 51, 0) (110, 51, 170) (110, 56, 160) (120, 56, 160) (120, 51, 170) (230, 51, 122.5) (220, 56, 122.5) (220, 56, 132.5) (230, 51, 37.5) (220, 56, 37.5) (220, 56, 47.5) (230, 51, 47.5) (230, 51, 132.5) (0, 51, 132.5) (10, 56, 132.5) (10, 56, 122.5) (0, 51, 47.5) (10, 56, 47.5) (10, 56, 37.5) (0, 51, 122.5) (0, 51, 37.5) on bodies 1
extrude "Extrude3" add sketch "Enclosure_upper" against normal blind 2 from surface at -3 contours L328 L330 L347 L351 | L328 L347 L351 L358 | L330 L347 L351 L360 | L347 L351 L356 L358 | L347 L351 L360 L362 | L343 L344 L347 A40 L348 L351 A44 L356 | L335 L346 A39 L347 L350 A43 L351 L362 | L341 L343 L344 L348 | L333 L335 L346 L350 | L341 L344 A37 L345 L348 A41 L349 L368 | L333 L345 A38 L346 L349 A42 L350 L366 | L345 L349 L368 L370 | L345 L349 L364 L366 | L336 L345 L349 L370 | L338 L345 L349 L364 | L336 L338 L345 L349 bodies 2
extrude "Extrude17" cut sketch "Enclosure_upper" against normal up to surface (3 mm away) contours A35 | A36 | A45 | A46 | A47 | A48 bodies 2
chamfer "Chamfer2" distance 3 angle 45 6 edges at (116.8647, 63, 5.7232) (116.8647, 63, 165.7232) (226.8647, 63, 43.2232) (226.8647, 63, 128.2232) (6.8647, 63, 43.2232) (6.8647, 63, 128.2232) on bodies 2
extrude "Extrude18" cut sketch "Enclosure_upper" against normal blind 2 from surface at -3 contours L347 L351 L356 L358 | L347 L356 L358 L359 | L351 L356 L357 L358 | L347 L360 L362 L363 | L347 L351 L360 L362 | L351 L360 L361 L362 | L340 L341 L343 L344 | L341 L343 L344 L348 | L341 L342 L343 L348 | L333 L335 L346 L350 | L333 L334 L335 L346 | L332 L333 L335 L350 | L345 L349 L368 L370 | L345 L368 L369 L370 | L349 L368 L370 L371 | L345 L364 L365 L366 | L345 L349 L364 L366 | L349 L364 L366 L367 bodies 2
fillet "Fillet6" radius 0.75 24 edges at (107.5, 59, 2) (107.5, 59, 0.5) (122.5, 59, 2) (122.5, 59, 0.5) (122.5, 59, 169.5) (122.5, 59, 168) (107.5, 59, 168) (107.5, 59, 169.5) (228, 59, 120) (229.5, 59, 120) (228, 59, 135) (229.5, 59, 135) (228, 59, 50) (229.5, 59, 50) (229.5, 59, 35) (228, 59, 35) (0.5, 59, 135) (2, 59, 135) (2, 59, 120) (0.5, 59, 120) (2, 59, 35) (0.5, 59, 35) (2, 59, 50) (0.5, 59, 50) on bodies 2
extrude "Extrude5" cut sketch "Enclosure_upper" against normal up to surface (3 mm away) contours A4 L47 L52 | A4 L43 L48 | A4 L51 L56 | A4 L39 L44 | A4 L55 | A4 L40 | A5 L40 | A5 L40 | A6 L40 | A6 L40 | A7 L55 | A7 L55 | A8 L55 | A8 L55 | A13 L61 | A9 L61 | A9 L61 | A12 L61 | A12 L61 | A13 L60 L65 | A13 L64 L69 | A13 L68 L73 | A13 L72 L77 | A13 L76 | A10 L76 | A10 L76 | A11 L76 | A11 L76 | A14 | A15 | A16 | A18 bodies 2
chamfer "Chamfer1" distance 3 angle 45 8 edges at (173.6147, 63, 58.9732) (216.1147, 63, 58.9732) (216.1147, 63, 16.4732) (173.6147, 63, 16.4732) (60.1147, 63, 58.9732) (60.1147, 63, 16.4732) (17.6147, 63, 16.4732) (17.6147, 63, 58.9732) on bodies 2
extrude "Extrude6" cut sketch "Enclosure_upper" against normal up to surface (3 mm away) contours L80 L81 L82 L83 | L93 L95 L134 L136 | L92 L93 L95 L134 | L93 L94 L95 L136 | L96 L97 L98 L99 | L141 L146 L175 L188 | L146 L166 L175 L188 | L146 L166 L173 L175 | L142 L195 L197 L198 | L169 L180 L183 L186 | L202 L223 L229 L238 | L202 L223 L229 L237 | L202 L223 L237 L250 | L203 L205 L213 L218 | L209 L222 L240 L247 | L264 L285 L291 L300 | L264 L285 L291 L299 | L264 L285 L299 L312 | L265 L267 L275 L280 | L271 L284 L302 L309 bodies 2
extrude "Extrude7" cut sketch "Enclosure_upper" along normal blind 1.5 from surface at -3 contours L86 L87 L89 L92 L93 L95 L134 | L89 L95 L134 L136 | L87 L93 L134 L136 | L87 L88 L89 L93 L94 L95 L136 | L114 L115 L116 L117 | L118 L119 L120 L121 | L122 L123 L124 L125 | L126 L127 L128 L129 | L130 L131 L132 L133 | L146 L166 L188 L189 | L141 L146 L175 L184 L188 L189 L191 | L146 L166 L173 L175 L185 L189 L191 | L166 L175 L188 L191 | L140 L143 L144 L159 | L147 L153 L156 L160 | L158 L174 L177 L194 | L162 L163 L196 L199 | L168 L170 L171 L176 | L201 L217 L219 L244 | L202 L221 L223 L224 L229 L238 L246 | L202 L224 L229 L237 | L202 L223 L224 L230 L237 L246 L250 | L223 L229 L237 L246 | L206 L207 L208 L257 | L211 L212 L225 L233 | L228 L251 L258 L261 | L252 L253 L254 L256 | L263 L279 L281 L306 | L264 L283 L285 L286 L291 L300 L308 | L264 L286 L291 L299 | L264 L285 L286 L292 L299 L308 L312 | L285 L291 L299 L308 | L268 L269 L270 L319 | L273 L274 L287 L295 | L290 L313 L320 L323 | L314 L315 L316 L318 bodies 2
extrude "Extrude8" add sketch "Enclosure_upper" against normal blind 2 from surface at -3 contours L86 L87 L89 L134 L352 L354 L355 | L89 L111 L134 L136 L354 | L87 L105 L134 L136 L352 | L87 L88 L89 L136 L352 L353 L354 | L108 L109 L110 L111 L134 L136 L137 L354 | L102 L103 L104 L105 L134 L135 L136 L352 | A19 | A20 | A21 | A22 | L138 L148 L149 L154 L155 L166 L178 L188 | L178 L179 L184 L188 L189 L190 L191 | L155 L166 L178 L188 L189 | L166 L172 L178 L185 L189 L190 L191 | L152 L166 L188 L190 L191 | L151 L152 L165 L166 L188 L190 L192 L193 | A23 | A24 | A25 | A26 | L216 L224 L229 L237 L255 | L216 L221 L224 L229 L232 L243 L246 | L216 L224 L230 L232 L237 L241 L246 | L229 L232 L237 L246 L249 | L204 L215 L216 L229 L231 L237 L255 L259 | L229 L232 L234 L235 L237 L245 L248 L249 | A27 | A28 | A29 | A30 | L278 L286 L291 L299 L317 | L278 L283 L286 L291 L294 L305 L308 | L278 L286 L292 L294 L299 L303 L308 | L291 L294 L299 L308 L311 | L266 L277 L278 L291 L293 L299 L317 L321 | L291 L294 L296 L297 L299 L307 L310 L311 | A31 | A32 | A33 | A34 bodies 2
extrude "Extrude9" cut sketch "Enclosure_upper" along normal blind 4.5 from surface at -5 contours A20 | A22 | A23 | A25 | A27 | A29 | A31 | A33 bodies 2
extrude "Extrude10" add sketch "Enclosure_upper" against normal blind 1 from surface at -1.5 contours L114 L115 L116 L117 | L118 L119 L120 L121 | L126 L127 L128 L129 | L130 L131 L132 L133 | L147 L153 L156 L160 | L158 L174 L177 L194 | L162 L163 L196 L199 | L168 L170 L171 L176 | L201 L217 L219 L244 | L211 L212 L225 L233 | L228 L251 L258 L261 | L252 L253 L254 L256 | L263 L279 L281 L306 | L273 L274 L287 L295 | L290 L313 L320 L323 | L314 L315 L316 L318 bodies 2
extrude "Extrude11" cut sketch "Enclosure_upper" along normal blind 0.5 from surface at -1.5 contours L122 L123 L124 L125 | L140 L143 L144 L159 | L206 L207 L208 L257 | L268 L269 L270 L319 bodies 2
extrude "Extrude12" add sketch "Enclosure_upper" against normal blind 1 from surface at -5 separate body contours L89 L95 L134 L136 | L89 L111 L134 L136 L354 | L87 L105 L134 L136 L352 | L87 L93 L134 L136 | L108 L109 L110 L111 L134 L136 L137 L354 | L93 L95 L134 L136 | L102 L103 L104 L105 L134 L135 L136 L352 makes body 3
fillet "Fillet2" radius 1 4 edges at (10.2, 57.5, 117.25) (10.2, 57.5, 125.05) (54.8, 57.5, 117.25) (54.8, 57.5, 125.05) on bodies 3
fillet "Fillet3" radius 0.5 80 edges at (47, 59, 125.05) (47, 59, 135.9) (54.8, 59, 125.05) (54.8, 59, 117.25) (18, 59, 135.9) (18, 59, 125.05) (10.2, 59, 125.05) (10.2, 59, 117.25) (18, 59, 117.25) (18, 59, 106.4) (47, 59, 106.4) (21.5, 62.25, 125.7) (21.5, 62.25, 112.7) (43.5, 62.25, 112.7) (43.5, 62.25, 125.7) (37.85, 61.5, 153.4) (37.85, 61.5, 140.7) (27.15, 61.5, 140.7) (27.15, 61.5, 153.4) (92.85, 61.5, 140.7) (82.15, 61.5, 140.7) (82.15, 61.5, 153.4) (92.85, 61.5, 153.4) (65.2, 59, 117.25) (65.2, 59, 125.05) (73, 59, 135.9) (73, 59, 117.25) (73, 59, 106.4) (102, 59, 106.4) (92.85, 61.5, 97.7) (82.15, 61.5, 97.7) (82.15, 61.5, 85) (92.85, 61.5, 85) (102, 59, 117.25) (109.8, 59, 117.25) (102, 59, 135.9) (102, 59, 125.05) (120.2, 59, 125.05) (128, 59, 135.9) (157, 59, 135.9) (157, 59, 125.05) (164.8, 59, 125.05) (164.8, 59, 117.25) (137.15, 61.5, 140.7) (147.85, 61.5, 140.7) (147.85, 61.5, 85) (120.2, 59, 117.25) (147.85, 61.5, 97.7) (128, 59, 117.25) (157, 59, 106.4) (147.85, 61.5, 153.4) (137.15, 61.5, 153.4) (137.15, 61.5, 97.7) (137.15, 61.5, 85) (27.15, 61.5, 85) (37.85, 61.5, 85) (37.85, 61.5, 97.7) (27.15, 61.5, 97.7) (109.8, 59, 125.05) (128, 59, 106.4) (183, 59, 106.4) (175.2, 59, 117.25) (183, 59, 117.25) (183, 59, 135.9) (202.85, 61.5, 153.4) (202.85, 61.5, 97.7) (192.15, 61.5, 97.7) (212, 59, 106.4) (212, 59, 117.25) (219.8, 59, 117.25) (219.8, 59, 125.05) (192.15, 61.5, 85) (202.85, 61.5, 85) (212, 59, 125.05) (212, 59, 135.9) (192.15, 61.5, 140.7) (202.85, 61.5, 140.7) (192.15, 61.5, 153.4) (175.2, 59, 125.05) (183, 59, 125.05) on bodies 2
extrude "Extrude13" add sketch "Enclosure_upper" against normal blind 7 from surface at -3 contours L324 L325 L326 L327 bodies 2
sketch "cable_holder" plane through (0, 0, 75.75) normal (0, 0, 1) x (1, 0, 0)
  line L0 (19, 60) -> (7, 60)
  line L1 (7, 60) -> (7, 53)
  line L2 (7, 53) -> (19, 53)
  line L3 (19, 53) -> (19, 60)
  line L4 (8, 59) -> (18, 59)
  line L5 (18, 59) -> (18, 54)
  line L6 (18, 54) -> (8, 54)
  line L7 (8, 54) -> (8, 59)
  line L8 (8, 56.5) -> (18, 56.5) construction
  line L9 (13, 59) -> (13, 54) construction
  line L10 (13, 60) -> (13, 53) construction
  line L11 (7, 56.5) -> (19, 56.5) construction
  dimension "d446" = 10
  dimension "d447" = 5
extrude "Extrude28" cut sketch "cable_holder" against normal up to surface (5 mm away) contours L4 L5 L6 L7 bodies 2
fillet "Fillet8" radius 2 8 edges at (19, 60, 73.25) (19, 53, 73.25) (7, 60, 73.25) (7, 53, 73.25) (18, 59, 73.25) (8, 59, 73.25) (18, 54, 73.25) (8, 54, 73.25) on bodies 2